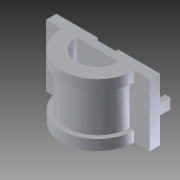
# Autodesk Inventor part: half_moon(hm)
Saved by Autodesk Inventor 2015 SP2 (Build 190223200, 223)
## iProperties
Created: 2015-12-12
Part Number: half_moon(hm)
Material: ABS Plastic
Document SubType Name: Modeling
Designer: elilitwack
Density: 1.06 g/cm^3
Appearance: Smooth - White
Author: elilitwack
Autodesk Inventor part; units mm, degrees
ref_plane "YZ Plane" through (0, 0, 0) normal (1, 0, 0) x (0, 1, 0)
ref_plane "XZ Plane" through (0, 0, 0) normal (0, 1, 0) x (-1, 0, 0)
ref_plane "XY Plane" through (0, 0, 0) normal (0, 0, 1) x (1, 0, 0)
sketch "base_sketch" plane through (0, 0, 0) normal (0, 0, 1) x (1, 0, 0)
  line L0 (0, 0) -> (50.8, 0)
  line L1 (50.8, 0) -> (50.8, 30.48)
  line L2 (50.8, 30.48) -> (0, 30.48)
  line L3 (0, 30.48) -> (0, 0)
  dimension "d0" = 50.8
  dimension "d1" = 30.48
  constraints: 8 end point, 2 parallel, 1 horizontal, 1 perpendicular
  measures "d0" distance of L1.end L2.end
  measures "d1" distance of L0.end L1.end
extrude "base_extrusion" add sketch "base_sketch" along normal blind 5.08
sketch "moon_sketch" plane through (0, 0, 5.08) normal (0, 0, 1) x (1, 0, 0)
  line L0 (0, 30.48) -> (0, 0) projected
  line L1 (0, 15.24) -> (25.4, 15.24) construction
  line L2 (25.4, 15.24) -> (50.8, 15.24) construction
  line L3 (25.4, 30.48) -> (25.4, 15.24)
  line L4 (0, 0) -> (50.8, 0) projected
  line L5 (25.4, 0) -> (25.4, 15.24)
  line L6 (50.8, 30.48) -> (0, 30.48) projected
  line L7 (25.4, 30.48) -> (43.18, 30.48)
  line L8 (43.18, 30.48) -> (43.18, 25.4)
  line L9 (43.18, 25.4) -> (40.894, 25.4)
  line L10 (40.894, 25.4) -> (40.894, 5.08)
  line L11 (40.894, 5.08) -> (43.18, 5.08)
  line L12 (43.18, 5.08) -> (43.18, 0)
  dimension "d4" = 17.78
  dimension "d5" = 5.08
  dimension "d6" = 2.286
  constraints: 20 end point, 6 perpendicular, 4 equal length, 3 midpoint, 3 point on line, 1 horizontal, 1 vertical
  measures "d4" distance of L3.start L7.end
  measures "d5" distance of L7.end L8.end
  measures "d6" distance of L8.end L9.end
revolve "moon_revolution" add sketch "moon_sketch" angle 180 about axis through (25.4, 30.48, 5.08) along (0, -1, 0) contours L6 L8 L9 L10 L11 L12 L4 L5 L3
sketch "cutout_sketch" plane through (0, 0, 0) normal (0, -1, 0) x (1, 0, 0)
  line L0 (43.18, 5.08) -> (7.62, 5.08)
  line L1 (42.8625, 5.08) -> (46.0375, 5.08) projected
  arc A0 (40.894, 5.08) -> (9.906, 5.08) centre (25.4, 5.08) ccw projected
  circle A1 centre (25.4, 5.08) radius 10.414
  line L2 (35.814, 5.08) -> (14.986, 5.08)
  point P0 (0, 0)
  point P1 (53.594, 5.08)
  point P2 (-2.794, 5.08)
  dimension "d16" = 5.08
  constraints: 4 end point, 2 point on circle, 1 centre point, 1 coincident, 1 collinear, 1 point on line, 1 other
extrude "cutout_extrusion" cut sketch "cutout_sketch" against normal up to next contours L0 A1 picked at (24.9454, 10.8279)
sketch "peg_sketch" plane through (0, 0, 0) normal (0, 0, -1) x (-1, 0, 0)
  line L0 (-50.8, 17.78) -> (-48.26, 17.78)
  line L1 (-48.26, 17.78) -> (-48.26, 12.7)
  line L2 (-48.26, 12.7) -> (-50.8, 12.7)
  line L3 (-50.8, 0) -> (-50.8, 30.48) projected
  line L4 (-50.8, 0) -> (-50.8, 12.7) construction
  line L5 (-50.8, 30.48) -> (-50.8, 17.78) construction
  line L6 (-50.8, 17.78) -> (-50.8, 12.7)
  line L7 (-2.54, 17.78) -> (0, 17.78)
  line L8 (0, 17.78) -> (0, 12.7)
  line L9 (0, 12.7) -> (-2.54, 12.7)
  line L10 (-2.54, 12.7) -> (-2.54, 17.78)
  line L11 (0, 30.48) -> (0, 17.78) construction
  line L12 (0, 12.7) -> (0, 0) construction
  line L13 (0, 30.48) -> (0, 0) construction
  dimension "d19" = 5.08
  dimension "d20" = 2.54
  dimension "d21" = 5.08
  dimension "d22" = 2.54
  constraints: 24 end point, 3 equal length, 3 perpendicular, 2 collinear, 2 horizontal, 2 parallel, 1 vertical
  measures "d19" distance of L0.end L1.end
  measures "d20" distance of L1.end L2.end
  measures "d21" distance of L9.end L7.start
  measures "d22" distance of L8.end L9.end
extrude "peg_extrusion" add sketch "peg_sketch" along normal blind 5.08
sketch "rivet_groove_sketch" plane through (0, 0, 0) normal (0, -1, 0) x (1, 0, 0)
  line L0 (20.32, 1.27) -> (30.48, 1.27)
  line L1 (30.48, 1.27) -> (30.48, 0)
  line L2 (30.48, 0) -> (20.32, 0)
  line L3 (20.32, 0) -> (20.32, 1.27)
  line L4 (50.8, 0) -> (30.48, 0) construction
  line L5 (0, 0) -> (20.32, 0) construction
  line L6 (50.8, 0) -> (50.8, 5.08) projected
  line L7 (0, 0) -> (50.8, 0) projected
  dimension "d25" = 10.16
  dimension "d26" = 1.27
  constraints: 12 end point, 2 collinear, 2 parallel, 1 horizontal, 1 perpendicular
  measures "d25" distance of L0.start L0.end
  measures "d26" distance of L0.end L1.end
extrude "rivet_groove_extrusion" cut sketch "rivet_groove_sketch" against normal up to next
equation "\"d0\" = hm_base_length"
equation "\"d1\" = hm_base_width"
equation "\"d2\" = hm_base_height"
equation "\"d4\" = hm_moon_flange_radius"
equation "\"d5\" = hm_moon_flange_width"
equation "\"d6\" = hm_moon_channel_offset"
equation "\"d16\" = hm_moon_thickness"
equation "\"d19\" = hm_peg_length"
equation "\"d20\" = hm_peg_width"
equation "\"d21\" = hm_peg_length"
equation "\"d22\" = hm_peg_width"
equation "\"d23\" = hm_peg_height"
equation "\"d25\" = hm_rivet_groove_width"
equation "\"d26\" = hm_rivet_groove_height"
equation "\"d27\" = hm_peg_height"
equation "\"hm_base_width\" = 30.48"
equation "\"hm_base_length\" = 50.8"
equation "\"hm_moon_flange_radius\" = 17.78"
equation "\"hm_moon_channel_offset\" = 2.286"
equation "\"hm_moon_flange_width\" = 5.08"
equation "\"hm_moon_thickness\" = 5.08"
equation "\"hm_peg_width\" = 2.54"
equation "\"hm_peg_length\" = 5.08"
equation "\"hm_base_height\" = 5.08"
equation "\"hm_peg_height\" = 5.08"
equation "\"hm_rivet_groove_width\" = 10.16"
equation "\"hm_rivet_groove_height\" = 1.27"
body "Solid1"
